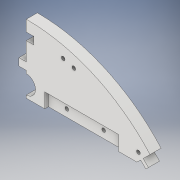
# Autodesk Inventor part: CP006
Saved by Autodesk Inventor 2017 SP1 (Build 210196100, 196)
## iProperties
Created: 2017-05-15
Part Number: CP006
Material: ABS Plastic
Document SubType Name: Modeling
Designer: zallen
Density: 1.06 g/cm^3
Appearance: Smooth - White
Mass: 171.786 g
Surface Area: 320.784 cm^2
Volume: 162.062 cm^3
Author: zallen
Autodesk Inventor part; units mm, degrees
ref_plane "YZ Plane" through (0, 0, 0) normal (1, 0, 0) x (0, 1, 0)
ref_plane "XZ Plane" through (0, 0, 0) normal (0, 1, 0) x (-1, 0, 0)
ref_plane "XY Plane" through (0, 0, 0) normal (0, 0, 1) x (1, 0, 0)
sketch "Sketch1" plane through (0, 0, 0) normal (0, 0, 1) x (1, 0, 0)
  circle A0 centre (0, -132.2876) radius 225 construction
  circle A1 centre (0, -132.2876) radius 200 construction
  line L0 (-225, -132.2876) -> (225, -132.2876) construction
  line L1 (150, -132.2876) -> (150, 35.4175) construction
  line L2 (175, -132.2876) -> (175, 9.1338) construction
  line L3 (0, 92.7124) -> (0, -357.2876) construction
  line L4 (150, 0) -> (0, 0)
  line L5 (0, 0) -> (0, 92.7124)
  line L6 (150, 0) -> (167.7086, 17.7086)
  line L7 (150, 0) -> (175.0437, 0) construction
  arc A2 (167.7086, 17.7086) -> (0, 92.7124) centre (0, -132.2876) ccw
  dimension "d0" = 450
  dimension "d1" = 25
  dimension "d2" = 75
  dimension "d3" = 25
  dimension "d4" = 45
  constraints: 16 end point, 4 midpoint, 4 point on line, 2 horizontal, 2 perpendicular, 2 point on circle, 2 vertical, 1 centre point, 1 coincident, 1 equal length, 1 parallel, 13 other
  measures "d2" distance of L1.start L0.end
  measures "d3" distance between parallel lines of L2 L1
  measures "d4" angle of L7 L6
extrude "Extrusion1" add sketch "Sketch1" along normal blind 15
sketch "Sketch2" plane through (0, 0, 15) normal (0, 0, 1) x (1, 0, 0)
  line L0 (10, 77.7124) -> (0, 77.7124)
  line L1 (0, 77.7124) -> (0, 67.7124)
  line L2 (0, 67.7124) -> (10, 67.7124)
  line L3 (10, 67.7124) -> (10, 77.7124)
  line L4 (0, 92.7124) -> (0, 0) projected
  line L5 (0, 0) -> (150, 0) projected
  line L6 (150, 0) -> (167.7086, 17.7086) projected
  arc A0 (167.7086, 17.7086) -> (0, 92.7124) centre (0, -132.2876) ccw projected
  line L7 (0, 92.7124) -> (0, 0) projected
  dimension "d7" = 10
  dimension "d8" = 10
  dimension "d21" = 15
  constraints: 8 end point, 2 parallel, 1 horizontal, 1 perpendicular, 1 point on line
  measures "d7" distance of L2.end L1.end
  measures "d8" distance of L1.end L0.end
  measures "d21" distance of L0.end L4.start
extrude "Extrusion2" cut sketch "Sketch2" against normal blind 15 contours L3 L2 L1 L0
sketch "Sketch3" plane through (0, 0, 15) normal (0, 0, 1) x (1, 0, 0)
  line L0 (-10, 42.7124) -> (0, 42.7124)
  line L1 (0, 42.7124) -> (0, 32.7124)
  line L2 (0, 32.7124) -> (-10, 32.7124)
  line L3 (-10, 32.7124) -> (-10, 42.7124)
  line L4 (0, 0) -> (150, 0) projected
  line L5 (150, 0) -> (167.7086, 17.7086) projected
  arc A0 (167.7086, 17.7086) -> (0, 92.7124) centre (0, -132.2876) ccw projected
  line L6 (0, 67.7124) -> (0, 0) projected
  line L7 (0, 67.7124) -> (0, 0) projected
  line L8 (10, 67.7124) -> (0, 67.7124) projected
  line L9 (0, 92.7124) -> (0, 77.7124) projected
  line L10 (0, 77.7124) -> (10, 77.7124) projected
  line L11 (10, 77.7124) -> (10, 67.7124) projected
  dimension "d15" = 10
  dimension "d16" = 10
  dimension "d20" = 25
  constraints: 8 end point, 2 parallel, 1 horizontal, 1 perpendicular, 1 point on line
  measures "d15" distance of L1.end L2.end
  measures "d16" distance of L0.end L1.end
  measures "d20" distance of L0.end L6.start
extrude "Extrusion3" add sketch "Sketch3" against normal blind 15 contours L0 L1 L2 L3
sketch "Sketch4" plane through (0, 0, 15) normal (0, 0, 1) x (1, 0, 0)
  line L0 (155, 5) -> (162.0711, -2.0711)
  line L1 (162.0711, -2.0711) -> (165.6066, 1.4645)
  line L2 (165.6066, 1.4645) -> (158.5355, 8.5355)
  line L3 (158.5355, 8.5355) -> (155, 5)
  line L4 (10, 67.7124) -> (0, 67.7124) projected
  line L5 (0, 67.7124) -> (0, 42.7124) projected
  line L6 (-10, 42.7124) -> (0, 42.7124) projected
  line L7 (-10, 32.7124) -> (-10, 42.7124) projected
  line L8 (0, 32.7124) -> (-10, 32.7124) projected
  line L9 (0, 32.7124) -> (0, 0) projected
  line L10 (0, 0) -> (150, 0) projected
  line L11 (150, 0) -> (167.7086, 17.7086) projected
  arc A0 (167.7086, 17.7086) -> (0, 92.7124) centre (0, -132.2876) ccw projected
  line L12 (0, 92.7124) -> (0, 77.7124) projected
  line L13 (0, 77.7124) -> (10, 77.7124) projected
  line L14 (10, 77.7124) -> (10, 67.7124) projected
  line L15 (150, 0) -> (167.7086, 17.7086) projected
  dimension "d22" = 10
  dimension "d23" = 5
  dimension "d24" = 5
  constraints: 8 end point, 2 parallel, 2 point on line, 1 perpendicular
  measures "d22" distance of L2.end L1.end
  measures "d23" distance of L1.end L0.end
  measures "d24" horizontal distance of L10.end L0.start
extrude "Extrusion4" add sketch "Sketch4" against normal blind 15 contours L3 L2 L1 L0
sketch "Sketch5" plane through (0, 0, 15) normal (0, 0, 1) x (1, 0, 0)
  line L0 (10, 67.7124) -> (0, 67.7124) construction
  line L1 (0, 67.7124) -> (0, 42.7124) construction
  line L2 (-10, 42.7124) -> (0, 42.7124) construction
  line L3 (-10, 32.7124) -> (-10, 42.7124) construction
  line L4 (0, 32.7124) -> (-10, 32.7124) construction
  line L5 (0, 32.7124) -> (0, 0) construction
  line L6 (0, 0) -> (150, 0) construction
  line L7 (150, 0) -> (155, 5) construction
  line L8 (155, 5) -> (162.0711, -2.0711) construction
  line L9 (162.0711, -2.0711) -> (165.6066, 1.4645) construction
  line L10 (165.6066, 1.4645) -> (158.5355, 8.5355) construction
  line L11 (158.5355, 8.5355) -> (167.7086, 17.7086) construction
  arc A0 (167.7086, 17.7086) -> (0, 92.7124) centre (0, -132.2876) ccw construction
  line L12 (0, 92.7124) -> (0, 77.7124) construction
  line L13 (0, 77.7124) -> (10, 77.7124) construction
  line L14 (10, 77.7124) -> (10, 67.7124) construction
  circle A1 centre (0, -132.2876) radius 225 construction
  arc A2 (167.7086, 17.7086) -> (0, 92.7124) centre (0, -132.2876) ccw construction
  circle A3 centre (0, -132.2876) radius 210 construction
  circle A4 centre (50, 71.6732) radius 2.5
  circle A5 centre (64.4318, 67.5838) radius 2.5
  circle A6 centre (152.0028, 12.6094) radius 2.5
  dimension "d27" = 450
  dimension "d28" = 15
  dimension "d31" = 5
  dimension "d32" = 5
  dimension "d33" = 15
  dimension "d34" = 50
  dimension "d46" = 5
  dimension "d49" = 7.5
  constraints: 5 centre point, 3 point on circle, 1 concentric
  measures "d27" diameter of A1
  measures "d28" radial gap between concentric circles of A1 A3
  measures "d31" diameter of A4
  measures "d32" diameter of A5
  measures "d33" distance of A5.centre A4.centre
  measures "d34" distance from line of L5 A4.centre
  measures "d46" diameter of A6
  measures "d49" distance from line of A6.centre L11
extrude "Extrusion5" cut sketch "Sketch5" against normal through all
thread "Thread1" size "M5x0.8" class "6H" standard "ANSI Metric M Profile" full length
thread "Thread2" size "M5x0.8" class "6H" standard "ANSI Metric M Profile" full length
thread "Thread4" size "M5x0.8" class "6H" standard "ANSI Metric M Profile" full length
sketch "Sketch7" plane through (0, 0, 15) normal (0, 0, 1) x (1, 0, 0)
  line L0 (0, 0) -> (150, 0) construction
  line L1 (25, 0) -> (125, 0) construction
  line L2 (125, 0) -> (125, 20) construction
  line L3 (125, 20) -> (25, 20) construction
  line L4 (25, 20) -> (25, 0) construction
  circle A0 centre (50, 10) radius 2.5
  circle A1 centre (100, 10) radius 2.5
  dimension "d52" = 100
  dimension "d53" = 20
  dimension "d54" = 25
  dimension "d55" = 5
  dimension "d56" = 5
  dimension "d57" = 25
  dimension "d58" = 25
  constraints: 8 end point, 2 centre point, 2 parallel, 1 horizontal, 1 perpendicular, 1 point on line
  measures "d52" distance of L3.end L2.end
  measures "d53" distance of L2.end L1.end
  measures "d54" distance of L0.start L1.start
  measures "d55" diameter of A0
  measures "d56" diameter of A1
  measures "d57" distance from line of L4 A0.centre
  measures "d58" distance from line of A1.centre L2
extrude "Extrusion6" cut sketch "Sketch7" against normal through all
thread "Thread5" size "M5x0.8" class "6H" standard "ANSI Metric M Profile" full length
thread "Thread6" size "M5x0.8" class "6H" standard "ANSI Metric M Profile" full length
sketch "Sketch8" plane through (0, 0, 15) normal (0, 0, 1) x (1, 0, 0)
  line L0 (0, 0) -> (150, 0) projected
  line L1 (25, 0) -> (125, 0)
  line L2 (125, 0) -> (125, 20)
  line L3 (125, 20) -> (25, 20)
  line L4 (25, 20) -> (25, 0)
  line L5 (0, 32.7124) -> (0, 0) projected
  dimension "d67" = 100
  dimension "d68" = 20
  dimension "d69" = 25
  constraints: 8 end point, 2 parallel, 1 horizontal, 1 perpendicular, 1 point on line
  measures "d67" distance of L3.end L2.end
  measures "d68" distance of L2.end L1.end
  measures "d69" distance between parallel lines of L5 L4
extrude "Extrusion7" cut sketch "Sketch8" against normal blind 5
sketch "Sketch9" plane through (0, 0, 15) normal (0, 0, 1) x (1, 0, 0)
  line L0 (0, 32.7124) -> (0, 0) projected
  circle A0 centre (0, 16.3562) radius 12.5
  dimension "d72" = 25
  constraints: 1 centre point, 1 midpoint
  measures "d72" diameter of A0
extrude "Extrusion8" cut sketch "Sketch9" against normal through all
sketch "Sketch10" plane through (0, 0, 0) normal (0, 0, -1) x (-1, 0, 0)
  circle A0 centre (-72, 9.4249) radius 2.5
  circle A1 centre (-88, 9.4249) radius 2.5
  point P0 (0, 0)
  dimension "d75" = 5
  dimension "d76" = 5
  dimension "d77" = 16
  dimension "d79" = 88
  dimension "d80" = 9.4249
  constraints: 2 centre point, 1 horizontal alignment
  measures "d75" diameter of A0
  measures "d76" diameter of A1
  measures "d77" distance of A1.centre A0.centre
  measures "d79" horizontal distance of point (0, 0) A1.centre
  measures "d80" vertical distance of A0.centre point (0, 0)
extrude "Extrusion9" cut sketch "Sketch10" against normal blind 5
thread "Thread8" size "M5x0.8" class "6H" standard "ANSI Metric M Profile" full length
thread "Thread9" size "M5x0.8" class "6H" standard "ANSI Metric M Profile" full length
equation "\"d35\" = d46"
body "Solid1"
